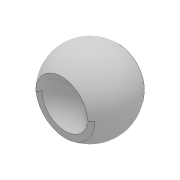
# Autodesk Inventor part: sensor_pad_small
Saved by Autodesk Inventor 2017 (Build 210142000, 142)
## iProperties
Created: 2018-05-30
Part Number: sensor_pad_small
Material: Generic
Document SubType Name: Modeling
Designer: Nic
Density: 1 g/cm^3
Appearance: Default
Author: Nic
Autodesk Inventor part; units mm, degrees
ref_plane "YZ Plane" through (0, 0, 0) normal (1, 0, 0) x (0, 1, 0)
ref_plane "XY Plane" through (0, 0, 0) normal (0, 0, 1) x (1, 0, 0)
sketch "Sketch1" plane through (0, 0, 0) normal (0, 0, 1) x (1, 0, 0)
  arc A0 (0, -14) -> (0, 14) centre (0, 0) ccw
  line L0 (0, 14) -> (0, -14)
  dimension "d0" = 28
  constraints: 2 end point, 2 point on circle, 1 centre point, 1 coincident, 1 midpoint, 1 vertical
  measures "d0" diameter of A0
revolve "Revolution1" add sketch "Sketch1" angle 360 about axis through (0, 14, 0) along (0, -1, 0)
sketch "Sketch2" plane through (0, 0, 0) normal (0, 0, 1) x (1, 0, 0)
  arc A0 (-11, 16) -> (11, 16) centre (0, 16) ccw
  line L0 (-11, 16) -> (11, 16)
  point P0 (0, 0)
  dimension "d2" = 16
  dimension "d19" = 22
  dimension "d20" = 11
  constraints: 2 end point, 2 point on circle, 1 centre point, 1 horizontal, 1 midpoint, 1 vertical alignment
  measures "d2" distance of point (0, 0) A0.centre
  measures "d19" distance of L0.start L0.end
  measures "d20" radius of A0
revolve "Revolution2" cut sketch "Sketch2" angle 360 about axis through (-11, 16, 0) along (1, 0, 0)
mirror "Mirror1" about plane through (0, 0, 0) normal (0, 1, 0) of "Revolution2"
ref_plane "Work Plane1" through (0, 9, 0) normal (0, 1, 0) x (-1, 0, 0)
sketch "Sketch3" plane through (0, 9, 0) normal (0, 1, 0) x (-1, 0, 0)
  line L0 (0, 0) -> (19, 0)
  line L1 (19, 0) -> (19, -16)
  line L2 (19, -16) -> (-19, -16)
  line L3 (-19, -16) -> (-19, 0)
  line L4 (-19, 0) -> (0, 0)
  line L5 (0, 0) -> (0, -16) construction
  dimension "d15" = 38
  dimension "d16" = 16
  constraints: 12 end point, 1 collinear, 1 horizontal, 1 midpoint, 1 parallel, 1 perpendicular, 1 point on line, 1 vertical, 1 other
  measures "d15" distance of L1.end L2.end
  measures "d16" distance of L2.end L3.end
extrude "Extrusion1" cut sketch "Sketch3" along normal blind 10
mirror "Mirror2" about plane through (0, 0, 0) normal (0, 1, 0) of "Extrusion1"
body "Solid1"
